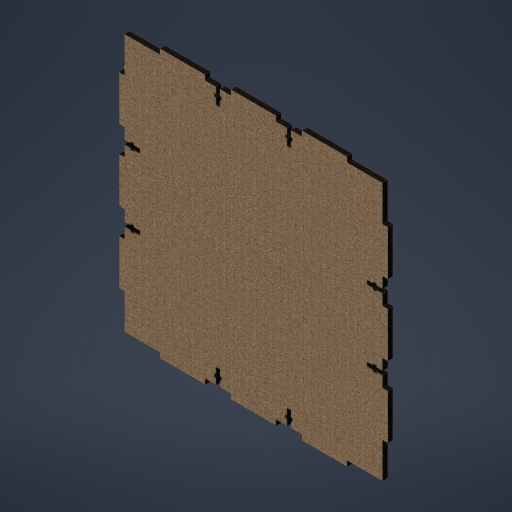
# Autodesk Inventor part: Floor
Saved by Autodesk Inventor 2024.1 (Build 281209000, 209)
## iProperties
Created: 2023-08-03
Part Number: Floor
Material: MDF Medium Density Fiberboard
Document SubType Name: Modeling
Designer: jaege
Density: 0.8 g/cm^3
Appearance: Cardboard - Corrugated
Author: jaege
Autodesk Inventor part; units mm, degrees
ref_plane "YZ Plane" through (0, 0, 0) normal (1, 0, 0) x (0, 1, 0)
ref_plane "XZ Plane" through (0, 0, 0) normal (0, 1, 0) x (-1, 0, 0)
ref_plane "XY Plane" through (0, 0, 0) normal (0, 0, 1) x (1, 0, 0)
ref_plane "Work Plane1" through (0, 0, 0) normal (0, 0, 1) x (1, 0, 0)
sketch "Sketch2" plane through (0, 0, 0) normal (0, 0, 1) x (1, 0, 0)
  line L0 (-4, -110) -> (-4, -145) projected
  line L1 (0, -110) -> (-4, -110) projected
  line L2 (0, -145) -> (0, -110) projected
  line L3 (0, -145) -> (-4, -145) projected
  line L4 (-4, -55) -> (-4, -90) projected
  line L5 (0, -55) -> (-4, -55) projected
  line L6 (0, -90) -> (0, -55) projected
  line L7 (0, -90) -> (-4, -90) projected
  line L8 (-4, 0) -> (-4, -35) projected
  line L9 (0, 0) -> (-4, 0) projected
  line L10 (0, -35) -> (0, 0) projected
  line L11 (0, -35) -> (-4, -35) projected
  line L12 (62.5, 31.5) -> (27.5, 31.5) projected
  line L13 (62.5, 27.5) -> (62.5, 31.5) projected
  line L14 (27.5, 27.5) -> (62.5, 27.5) projected
  line L15 (27.5, 27.5) -> (27.5, 31.5) projected
  line L16 (117.5, 31.5) -> (82.5, 31.5) projected
  line L17 (117.5, 27.5) -> (117.5, 31.5) projected
  line L18 (82.5, 27.5) -> (117.5, 27.5) projected
  line L19 (82.5, 27.5) -> (82.5, 31.5) projected
  line L20 (172.5, 31.5) -> (137.5, 31.5) projected
  line L21 (172.5, 27.5) -> (172.5, 31.5) projected
  line L22 (137.5, 27.5) -> (172.5, 27.5) projected
  line L23 (137.5, 27.5) -> (137.5, 31.5) projected
  line L24 (204, -35) -> (204, 0) projected
  line L25 (200, -35) -> (204, -35) projected
  line L26 (200, 0) -> (200, -35) projected
  line L27 (200, 0) -> (204, 0) projected
  line L28 (204, -90) -> (204, -55) projected
  line L29 (200, -90) -> (204, -90) projected
  line L30 (200, -55) -> (200, -90) projected
  line L31 (200, -55) -> (204, -55) projected
  line L32 (204, -145) -> (204, -110) projected
  line L33 (200, -145) -> (204, -145) projected
  line L34 (200, -110) -> (200, -145) projected
  line L35 (200, -110) -> (204, -110) projected
  line L36 (137.5, -176.5) -> (172.5, -176.5) projected
  line L37 (137.5, -172.5) -> (137.5, -176.5) projected
  line L38 (172.5, -172.5) -> (137.5, -172.5) projected
  line L39 (172.5, -172.5) -> (172.5, -176.5) projected
  line L40 (82.5, -176.5) -> (117.5, -176.5) projected
  line L41 (82.5, -172.5) -> (82.5, -176.5) projected
  line L42 (117.5, -172.5) -> (82.5, -172.5) projected
  line L43 (117.5, -172.5) -> (117.5, -176.5) projected
  line L44 (27.5, -176.5) -> (62.5, -176.5) projected
  line L45 (27.5, -172.5) -> (27.5, -176.5) projected
  line L46 (62.5, -172.5) -> (27.5, -172.5) projected
  line L47 (62.5, -172.5) -> (62.5, -176.5) projected
  line L48 (0, -172.5) -> (200, -172.5)
  line L49 (200, -172.5) -> (200, 27.5)
  line L50 (200, 27.5) -> (0, 27.5)
  line L51 (0, 27.5) -> (0, -172.5)
  point P0 (0, 27.5)
  point P1 (200, -172.5)
  constraints: 8 end point, 2 parallel, 1 horizontal, 1 perpendicular, 4 other
extrude "Extrusion2" add sketch "Sketch2" along normal blind 4
sketch "Sketch3" plane through (0, 0, 4) normal (0, 0, 1) x (1, 0, 0)
  line L0 (71, 27.5) -> (74, 27.5)
  line L1 (74, 27.5) -> (74, 15.5)
  line L2 (74, 15.5) -> (71, 15.5)
  line L3 (71, 15.5) -> (71, 27.5)
  line L4 (69.8, 22.7) -> (75.2, 22.7)
  line L5 (75.2, 22.7) -> (75.2, 20.3)
  line L6 (75.2, 20.3) -> (69.8, 20.3)
  line L7 (69.8, 20.3) -> (69.8, 22.7)
  line L8 (124.8, 22.7) -> (130.2, 22.7)
  line L9 (130.2, 22.7) -> (130.2, 20.3)
  line L10 (130.2, 20.3) -> (124.8, 20.3)
  line L11 (124.8, 20.3) -> (124.8, 22.7)
  line L12 (126, 27.5) -> (129, 27.5)
  line L13 (129, 27.5) -> (129, 15.5)
  line L14 (129, 15.5) -> (126, 15.5)
  line L15 (126, 15.5) -> (126, 27.5)
  line L16 (-4, -145) -> (0, -145) projected
  line L17 (0, -145) -> (0, -172.5) projected
  line L18 (0, -172.5) -> (27.5, -172.5) projected
  line L19 (27.5, -172.5) -> (27.5, -176.5) projected
  line L20 (27.5, -176.5) -> (62.5, -176.5) projected
  line L21 (62.5, -176.5) -> (62.5, -172.5) projected
  line L22 (62.5, -172.5) -> (82.5, -172.5) projected
  line L23 (82.5, -172.5) -> (82.5, -176.5) projected
  line L24 (82.5, -176.5) -> (117.5, -176.5) projected
  line L25 (117.5, -176.5) -> (117.5, -172.5) projected
  line L26 (117.5, -172.5) -> (137.5, -172.5) projected
  line L27 (137.5, -172.5) -> (137.5, -176.5) projected
  line L28 (137.5, -176.5) -> (172.5, -176.5) projected
  line L29 (172.5, -176.5) -> (172.5, -172.5) projected
  line L30 (172.5, -172.5) -> (200, -172.5) projected
  line L31 (200, -172.5) -> (200, -145) projected
  line L32 (200, -145) -> (204, -145) projected
  line L33 (204, -145) -> (204, -110) projected
  line L34 (204, -110) -> (200, -110) projected
  line L35 (200, -110) -> (200, -90) projected
  line L36 (200, -90) -> (204, -90) projected
  line L37 (204, -90) -> (204, -55) projected
  line L38 (204, -55) -> (200, -55) projected
  line L39 (200, -55) -> (200, -35) projected
  line L40 (200, -35) -> (204, -35) projected
  line L41 (204, -35) -> (204, 0) projected
  line L42 (204, 0) -> (200, 0) projected
  line L43 (200, 0) -> (200, 27.5) projected
  line L44 (200, 27.5) -> (172.5, 27.5) projected
  line L45 (172.5, 27.5) -> (172.5, 31.5) projected
  line L46 (172.5, 31.5) -> (137.5, 31.5) projected
  line L47 (137.5, 31.5) -> (137.5, 27.5) projected
  line L48 (137.5, 27.5) -> (117.5, 27.5) projected
  line L49 (117.5, 27.5) -> (117.5, 31.5) projected
  line L50 (117.5, 31.5) -> (82.5, 31.5) projected
  line L51 (82.5, 31.5) -> (82.5, 27.5) projected
  line L52 (82.5, 27.5) -> (62.5, 27.5) projected
  line L53 (62.5, 27.5) -> (62.5, 31.5) projected
  line L54 (62.5, 31.5) -> (27.5, 31.5) projected
  line L55 (27.5, 31.5) -> (27.5, 27.5) projected
  line L56 (27.5, 27.5) -> (0, 27.5) projected
  line L57 (0, 27.5) -> (0, 0) projected
  line L58 (0, 0) -> (-4, 0) projected
  line L59 (-4, 0) -> (-4, -35) projected
  line L60 (-4, -35) -> (0, -35) projected
  line L61 (0, -35) -> (0, -55) projected
  line L62 (0, -55) -> (-4, -55) projected
  line L63 (-4, -55) -> (-4, -90) projected
  line L64 (-4, -90) -> (0, -90) projected
  line L65 (0, -90) -> (0, -110) projected
  line L66 (0, -110) -> (-4, -110) projected
  line L67 (-4, -110) -> (-4, -145) projected
  line L68 (137.5, 27.5) -> (117.5, 27.5) projected
  line L69 (27.5, 27.5) -> (0, 27.5) projected
  line L70 (0, 27.5) -> (200, -172.5) construction
  line L71 (0, -101.5) -> (0, -98.5)
  line L72 (0, -98.5) -> (12, -98.5)
  line L73 (12, -98.5) -> (12, -101.5)
  line L74 (12, -101.5) -> (0, -101.5)
  line L75 (4.8, -102.7) -> (4.8, -97.3)
  line L76 (4.8, -97.3) -> (7.2, -97.3)
  line L77 (7.2, -97.3) -> (7.2, -102.7)
  line L78 (7.2, -102.7) -> (4.8, -102.7)
  line L79 (12, -43.5) -> (12, -46.5)
  line L80 (7.2, -47.7) -> (4.8, -47.7)
  line L81 (7.2, -42.3) -> (7.2, -47.7)
  line L82 (4.8, -47.7) -> (4.8, -42.3)
  line L83 (12, -46.5) -> (0, -46.5)
  line L84 (0, -43.5) -> (12, -43.5)
  line L85 (0, -46.5) -> (0, -43.5)
  line L86 (4.8, -42.3) -> (7.2, -42.3)
  line L87 (129, -172.5) -> (126, -172.5)
  line L88 (126, -172.5) -> (126, -160.5)
  line L89 (126, -160.5) -> (129, -160.5)
  line L90 (129, -160.5) -> (129, -172.5)
  line L91 (130.2, -167.7) -> (124.8, -167.7)
  line L92 (124.8, -167.7) -> (124.8, -165.3)
  line L93 (124.8, -165.3) -> (130.2, -165.3)
  line L94 (130.2, -165.3) -> (130.2, -167.7)
  line L95 (71, -160.5) -> (74, -160.5)
  line L96 (75.2, -165.3) -> (75.2, -167.7)
  line L97 (69.8, -165.3) -> (75.2, -165.3)
  line L98 (75.2, -167.7) -> (69.8, -167.7)
  line L99 (74, -160.5) -> (74, -172.5)
  line L100 (71, -172.5) -> (71, -160.5)
  line L101 (74, -172.5) -> (71, -172.5)
  line L102 (69.8, -167.7) -> (69.8, -165.3)
  line L103 (200, -43.5) -> (200, -46.5)
  line L104 (200, -46.5) -> (188, -46.5)
  line L105 (188, -46.5) -> (188, -43.5)
  line L106 (188, -43.5) -> (200, -43.5)
  line L107 (195.2, -42.3) -> (195.2, -47.7)
  line L108 (195.2, -47.7) -> (192.8, -47.7)
  line L109 (192.8, -47.7) -> (192.8, -42.3)
  line L110 (192.8, -42.3) -> (195.2, -42.3)
  line L111 (188, -101.5) -> (188, -98.5)
  line L112 (192.8, -97.3) -> (195.2, -97.3)
  line L113 (192.8, -102.7) -> (192.8, -97.3)
  line L114 (195.2, -97.3) -> (195.2, -102.7)
  line L115 (188, -98.5) -> (200, -98.5)
  line L116 (200, -101.5) -> (188, -101.5)
  line L117 (200, -98.5) -> (200, -101.5)
  line L118 (195.2, -102.7) -> (192.8, -102.7)
  point P0 (72.5, 15.5)
  point P1 (72.5, 20.3)
  point P2 (72.5, 27.5)
  point P3 (127.5, 27.5)
  point P4 (127.5, 22.7)
  point P5 (127.5, 15.5)
  point P6 (127.5, 27.5)
  point P7 (127.5, 20.3)
  point P8 (75.2, 21.5)
  point P9 (74, 21.5)
  point P10 (100, -72.5)
  point P11 (6, -98.5)
  point P12 (12, -100)
  point P13 (6, -97.3)
  point P14 (7.2, -100)
  point P15 (0, -100)
  point P16 (12, -45)
  point P17 (7.2, -45)
  point P18 (4.8, -45)
  point P19 (0, -45)
  point P20 (0, -45)
  point P21 (126, -166.5)
  point P22 (127.5, -160.5)
  point P23 (124.8, -166.5)
  point P24 (127.5, -165.3)
  point P25 (127.5, -172.5)
  point P26 (72.5, -160.5)
  point P27 (72.5, -165.3)
  point P28 (72.5, -167.7)
  point P29 (72.5, -172.5)
  point P30 (72.5, -172.5)
  point P31 (194, -46.5)
  point P32 (188, -45)
  point P33 (194, -47.7)
  point P34 (192.8, -45)
  point P35 (200, -45)
  point P36 (188, -100)
  point P37 (192.8, -100)
  point P38 (195.2, -100)
  point P39 (200, -100)
  point P40 (200, -100)
  point P41 (4.8, -46.5)
  point P42 (7.2, -46.5)
  point P43 (7.2, -43.5)
  point P44 (4.8, -43.5)
  point P45 (74, 22.7)
  point P46 (71, 22.7)
  point P47 (71, 20.3)
  point P48 (74, 20.3)
  point P49 (195.2, -46.5)
  point P50 (195.2, -43.5)
  point P51 (192.8, -43.5)
  point P52 (192.8, -46.5)
  point P53 (126, 22.7)
  point P54 (126, 20.3)
  point P55 (129, 20.3)
  point P56 (129, 22.7)
  point P57 (74, -167.7)
  point P58 (74, -165.3)
  point P59 (71, -165.3)
  point P60 (71, -167.7)
  point P61 (4.8, -98.5)
  point P62 (4.8, -101.5)
  point P63 (7.2, -101.5)
  point P64 (7.2, -98.5)
  point P65 (195.2, -98.5)
  point P66 (192.8, -98.5)
  point P67 (192.8, -101.5)
  point P68 (195.2, -101.5)
  point P69 (126, -167.7)
  point P70 (129, -167.7)
  point P71 (129, -165.3)
  point P72 (126, -165.3)
  dimension "d4" = 3
  dimension "d5" = 12
  dimension "d6" = 2.4
  dimension "d7" = 5.4
  dimension "d10" = 360
  constraints: 130 end point, 11 midpoint, 8 parallel, 8 point on line, 4 equal length, 4 horizontal, 4 perpendicular, 4 vertical alignment, 3 horizontal alignment, 169 other
  measures "d4" distance of L1.end L2.end
  measures "d5" distance of L0.end L1.end
  measures "d6" distance of L6.end L4.start
  measures "d7" distance of L5.end L6.end
extrude "Extrusion3" cut sketch "Sketch3" against normal up to next contours L0 L1 L4 L3 | L4 L1 L6 L3 | L3 L6 L7 L4 | L4 L5 L6 L1 | L6 L1 L2 L3 | L12 L13 L8 L15 | L15 L10 L11 L8 | L8 L13 L10 L15 | L8 L9 L10 L13 | L10 L13 L14 L15 | L84 L82 L83 L61 | L84 L81 L83 L82 | L82 L86 L81 L84 | L83 L81 L80 L82 | L84 L79 L83 L81 | L72 L75 L74 L65 | L39 L104 L107 L106 | L75 L76 L77 L72 | L72 L77 L74 L75 | L107 L104 L109 L106 | L106 L109 L110 L107 | L74 L77 L78 L75 | L72 L73 L74 L77 | L107 L108 L109 L104 | L109 L104 L105 L106 | L35 L116 L114 L115 | L115 L113 L112 L114 | L114 L116 L113 L115 | L114 L118 L113 L116 | L113 L116 L111 L115 | L100 L98 L99 L22 | L100 L97 L99 L98 | L98 L102 L97 L100 | L99 L97 L96 L98 | L100 L95 L99 L97 | L88 L91 L90 L26 | L91 L92 L93 L88 | L88 L93 L90 L91 | L90 L93 L94 L91 | L88 L89 L90 L93
body "Solid2"
